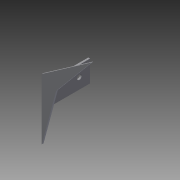
# Autodesk Inventor part: Left Hip
Saved by Autodesk Inventor 2014 (Build 180170000, 170)
## iProperties
Created: 2015-08-01
Part Number: Left Hip
Material: Generic
Document SubType Name: Modeling
Designer: Devon
Density: 1 g/cm^3
Appearance: Default
Author: Devon
Autodesk Inventor part; units mm, degrees
ref_plane "YZ Plane" through (0, 0, 0) normal (1, 0, 0) x (0, 1, 0)
ref_plane "XZ Plane" through (0, 0, 0) normal (0, 1, 0) x (-1, 0, 0)
ref_plane "XY Plane" through (0, 0, 0) normal (0, 0, 1) x (1, 0, 0)
sketch "Sketch1" plane through (0, 0, 0) normal (0, 0, 1) x (1, 0, 0)
  line L0 (2.2943, 2.9258) -> (2.2943, -105.0242)
  line L1 (2.2943, 2.9258) -> (90.7218, 64.8434)
  line L2 (90.7218, 64.8434) -> (27.6787, -10.2885)
  line L3 (2.2943, -105.0242) -> (27.6787, -10.2885)
  point P0 (0, 0)
  dimension "d0" = 107.95
  dimension "d1" = 107.95
  constraints: 8 end point, 1 vertical
  measures "d0" distance of L0.start L0.end
  measures "d1" distance of L0.start L1.end
extrude "Extrusion1" add sketch "Sketch1" along normal blind 3.175
sketch "Sketch2" plane through (0, 0, 0) normal (0, 0, -1) x (-1, 0, 0)
  line L0 (-2.2943, 2.9258) -> (-2.2943, -105.0242)
  line L1 (-2.2943, -51.0492) -> (-5.4693, -51.0492)
  line L2 (-5.4693, -51.0492) -> (-5.4693, -12.9492)
  line L3 (-5.4693, -12.9492) -> (-2.2943, -12.9492)
  point P0 (0, 0)
  dimension "d8" = 3.175
  dimension "d9" = 38.1
  constraints: 8 end point, 1 midpoint, 1 perpendicular, 1 point on line
  measures "d8" distance of L1.start L1.end
  measures "d9" distance of L1.end L2.end
extrude "Extrusion2" add sketch "Sketch2" along normal blind 79.2734
sketch "Sketch3" plane through (2.2943, -105.0242, 3.175) normal (-1, 0, 0) x (0, 0, 1)
  line L0 (-82.4484, 92.075) -> (-63.3984, 92.075)
  line L1 (-63.3984, 92.075) -> (-63.3984, 73.025)
  line L2 (-63.3984, 73.025) -> (-82.4484, 73.025)
  line L3 (-82.4484, 73.025) -> (-82.4484, 92.075)
  point P0 (-3.175, 105.0242)
  dimension "d12" = 19.05
  dimension "d13" = 19.05
  constraints: 8 end point, 2 parallel, 1 horizontal, 1 perpendicular
  measures "d12" distance of L1.end L2.end
  measures "d13" distance of L0.end L1.end
hole "Hole1" at (2.2943, -31.9992, -60.2234) direction (1, 0, 0) diameter 8.3312 end through all
body "Solid1"
